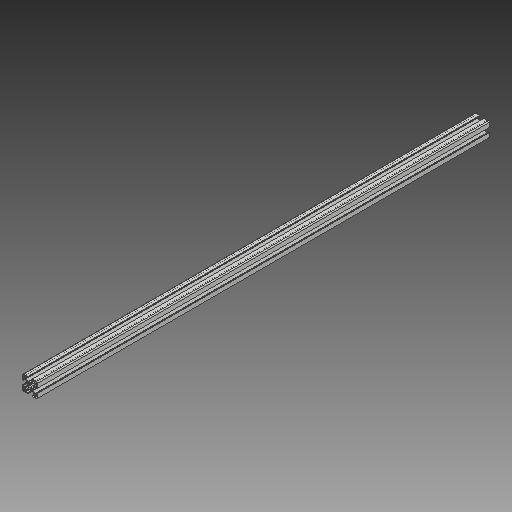
# Autodesk Inventor part: 3030 900mm_CPY
Saved by Autodesk Inventor 2018 (Build 220112000, 112)
## iProperties
Created: 2016-07-11
Part Number: 3030 900mm_CPY
Material: Generic
Document SubType Name: Modeling
Designer: joshmamo
Density: 1 g/cm^3
Appearance: Default
Author: joshm
Autodesk Inventor part; units mm, degrees
ref_plane "YZ Plane" through (0, 0, 0) normal (1, 0, 0) x (0, 1, 0)
ref_plane "XZ Plane" through (0, 0, 0) normal (0, 1, 0) x (-1, 0, 0)
ref_plane "XY Plane" through (0, 0, 0) normal (0, 0, 1) x (1, 0, 0)
sketch "Sketch1" plane through (0, 0, 0) normal (0, 0, 1) x (1, 0, 0)
  line L0 (-2.4733, -3.9798) -> (-1.4942, -3.198) projected
  arc A0 (-1.4942, -3.198) -> (1.4942, -3.198) centre (0, 0.0001) ccw projected
  line L1 (1.4942, -3.198) -> (2.4733, -3.9798) projected
  arc A1 (2.4733, -3.9798) -> (3.9799, -2.4732) centre (3.1422, -3.1421) ccw projected
  line L2 (3.9799, -2.4732) -> (3.1981, -1.4941) projected
  arc A2 (3.1981, -1.4941) -> (3.1981, 1.4944) centre (0, 0.0001) ccw projected
  line L3 (3.1981, 1.4944) -> (3.9799, 2.4735) projected
  arc A3 (3.9799, 2.4735) -> (2.4733, 3.9801) centre (3.1422, 3.1424) ccw projected
  line L4 (2.4733, 3.9801) -> (1.4942, 3.1983) projected
  arc A4 (1.4942, 3.1983) -> (-1.4942, 3.1983) centre (0, 0.0001) ccw projected
  line L5 (-1.4942, 3.1983) -> (-2.4733, 3.9801) projected
  arc A5 (-2.4733, 3.9801) -> (-3.9799, 2.4735) centre (-3.1422, 3.1424) ccw projected
  line L6 (-3.9799, 2.4735) -> (-3.1981, 1.4944) projected
  arc A6 (-3.1981, 1.4944) -> (-3.1981, -1.4941) centre (0, 0.0001) ccw projected
  line L7 (-3.1981, -1.4941) -> (-3.9799, -2.4732) projected
  arc A7 (-3.9799, -2.4732) -> (-2.4733, -3.9798) centre (-3.1422, -3.1421) ccw projected
  line L8 (13.3189, -9.4998) -> (9.88, -9.4998) projected
  arc A8 (9.88, -9.4998) -> (9.5, -9.8798) centre (9.88, -9.8798) ccw projected
  line L9 (9.5, -9.8798) -> (9.5, -13.3188) projected
  arc A9 (9.5, -13.3188) -> (9.881, -13.6998) centre (9.881, -13.3188) ccw projected
  line L10 (9.881, -13.6998) -> (12.6999, -13.6998) projected
  arc A10 (12.6999, -13.6998) -> (13.6999, -12.6998) centre (12.6999, -12.6998) ccw projected
  line L11 (13.6999, -12.6998) -> (13.6999, -9.8808) projected
  arc A11 (13.6999, -9.8808) -> (13.3189, -9.4998) centre (13.3189, -9.8808) ccw projected
  line L12 (-9.5, -13.3188) -> (-9.5, -9.8798) projected
  arc A12 (-9.5, -9.8798) -> (-9.88, -9.4998) centre (-9.88, -9.8798) ccw projected
  line L13 (-9.88, -9.4998) -> (-13.3189, -9.4998) projected
  arc A13 (-13.3189, -9.4998) -> (-13.6999, -9.8808) centre (-13.3189, -9.8808) ccw projected
  line L14 (-13.6999, -9.8808) -> (-13.6999, -12.6998) projected
  arc A14 (-13.6999, -12.6998) -> (-12.6999, -13.6998) centre (-12.6999, -12.6998) ccw projected
  line L15 (-12.6999, -13.6998) -> (-9.881, -13.6998) projected
  arc A15 (-9.881, -13.6998) -> (-9.5, -13.3188) centre (-9.881, -13.3188) ccw projected
  line L16 (-13.3189, 9.5001) -> (-9.88, 9.5001) projected
  arc A16 (-9.88, 9.5001) -> (-9.5, 9.8801) centre (-9.88, 9.8801) ccw projected
  line L17 (-9.5, 9.8801) -> (-9.5, 13.3191) projected
  arc A17 (-9.5, 13.3191) -> (-9.881, 13.7001) centre (-9.881, 13.3191) ccw projected
  line L18 (-9.881, 13.7001) -> (-12.6999, 13.7001) projected
  arc A18 (-12.6999, 13.7001) -> (-13.6999, 12.7001) centre (-12.6999, 12.7001) ccw projected
  line L19 (-13.6999, 12.7001) -> (-13.6999, 9.8811) projected
  arc A19 (-13.6999, 9.8811) -> (-13.3189, 9.5001) centre (-13.3189, 9.8811) ccw projected
  line L20 (9.5, 13.3191) -> (9.5, 9.8801) projected
  arc A20 (9.5, 9.8801) -> (9.88, 9.5001) centre (9.88, 9.8801) ccw projected
  line L21 (9.88, 9.5001) -> (13.3189, 9.5001) projected
  arc A21 (13.3189, 9.5001) -> (13.6999, 9.8811) centre (13.3189, 9.8811) ccw projected
  line L22 (13.6999, 9.8811) -> (13.6999, 12.7001) projected
  arc A22 (13.6999, 12.7001) -> (12.6999, 13.7001) centre (12.6999, 12.7001) ccw projected
  line L23 (12.6999, 13.7001) -> (9.881, 13.7001) projected
  arc A23 (9.881, 13.7001) -> (9.5, 13.3191) centre (9.881, 13.3191) ccw projected
  arc A24 (4, 13.2426) -> (4.5, 12.7426) centre (4.5, 13.2426) ccw projected
  line L24 (4, 13.2426) -> (4, 14.5001) projected
  arc A25 (4.5, 15.0001) -> (4, 14.5001) centre (4.5, 14.5001) ccw projected
  line L25 (4.5, 15.0001) -> (12.9999, 15.0001) projected
  arc A26 (14.9999, 13.0001) -> (12.9999, 15.0001) centre (12.9999, 13.0001) ccw projected
  line L26 (14.9999, 13.0001) -> (14.9999, 4.5001) projected
  arc A27 (14.4999, 4.0001) -> (14.9999, 4.5001) centre (14.4999, 4.5001) ccw projected
  line L27 (14.4999, 4.0001) -> (13.2425, 4.0001) projected
  arc A28 (12.7425, 4.5001) -> (13.2425, 4.0001) centre (13.2425, 4.5001) ccw projected
  line L28 (12.7425, 4.5001) -> (12.7425, 7.7327) projected
  arc A29 (12.7425, 7.7327) -> (12.2428, 8.2501) centre (12.2428, 7.7501) ccw projected
  line L29 (12.2428, 8.2501) -> (10.2602, 8.2501) projected
  arc A30 (10.2602, 8.2501) -> (9.9066, 8.1037) centre (10.2602, 7.7501) ccw projected
  line L30 (9.9066, 8.1037) -> (5.9811, 4.1781) projected
  arc A31 (5.9811, 4.1781) -> (5.8347, 3.8246) centre (6.3347, 3.8246) ccw projected
  line L31 (5.8347, 3.8246) -> (5.8347, 0.8876) projected
  line L32 (5.8347, 0.8876) -> (5.3247, -0.0624) projected
  line L33 (5.3247, -0.0624) -> (5.8347, -1.0124) projected
  line L34 (5.8347, -1.0124) -> (5.8347, -3.8243) projected
  arc A32 (5.8347, -3.8243) -> (5.9811, -4.1779) centre (6.3347, -3.8243) ccw projected
  line L35 (5.9811, -4.1779) -> (9.9066, -8.1034) projected
  arc A33 (9.9066, -8.1034) -> (10.2602, -8.2498) centre (10.2602, -7.7498) ccw projected
  line L36 (10.2602, -8.2498) -> (12.2428, -8.2498) projected
  arc A34 (12.2428, -8.2498) -> (12.7425, -7.7324) centre (12.2428, -7.7498) ccw projected
  line L37 (12.7425, -7.7324) -> (12.7425, -4.4999) projected
  arc A35 (13.2425, -3.9999) -> (12.7425, -4.4999) centre (13.2425, -4.4999) ccw projected
  line L38 (13.2425, -3.9999) -> (14.4999, -3.9999) projected
  arc A36 (14.9999, -4.4999) -> (14.4999, -3.9999) centre (14.4999, -4.4999) ccw projected
  line L39 (14.9999, -4.4999) -> (14.9999, -12.9998) projected
  arc A37 (12.9999, -14.9998) -> (14.9999, -12.9998) centre (12.9999, -12.9998) ccw projected
  line L40 (12.9999, -14.9998) -> (4.5, -14.9998) projected
  arc A38 (4, -14.4998) -> (4.5, -14.9998) centre (4.5, -14.4998) ccw projected
  line L41 (4, -14.4998) -> (4, -13.2423) projected
  arc A39 (4.5, -12.7423) -> (4, -13.2423) centre (4.5, -13.2423) ccw projected
  line L42 (4.5, -12.7423) -> (7.7325, -12.7423) projected
  arc A40 (7.7325, -12.7423) -> (8.25, -12.2426) centre (7.75, -12.2426) ccw projected
  line L43 (8.25, -12.2426) -> (8.25, -10.26) projected
  arc A41 (8.25, -10.26) -> (8.1035, -9.9065) centre (7.75, -10.26) ccw projected
  line L44 (8.1035, -9.9065) -> (4.178, -5.981) projected
  arc A42 (4.178, -5.981) -> (3.8245, -5.8345) centre (3.8245, -6.3345) ccw projected
  line L45 (3.8245, -5.8345) -> (0.95, -5.8345) projected
  line L46 (0.95, -5.8345) -> (0, -5.3245) projected
  line L47 (0, -5.3245) -> (-0.95, -5.8345) projected
  line L48 (-0.95, -5.8345) -> (-3.8245, -5.8345) projected
  arc A43 (-3.8245, -5.8345) -> (-4.178, -5.981) centre (-3.8245, -6.3345) ccw projected
  line L49 (-4.178, -5.981) -> (-8.1035, -9.9065) projected
  arc A44 (-8.1035, -9.9065) -> (-8.25, -10.26) centre (-7.75, -10.26) ccw projected
  line L50 (-8.25, -10.26) -> (-8.25, -12.2426) projected
  arc A45 (-8.25, -12.2426) -> (-7.7325, -12.7423) centre (-7.75, -12.2426) ccw projected
  line L51 (-7.7325, -12.7423) -> (-4.5, -12.7423) projected
  arc A46 (-4, -13.2423) -> (-4.5, -12.7423) centre (-4.5, -13.2423) ccw projected
  line L52 (-4, -13.2423) -> (-4, -14.4998) projected
  arc A47 (-4.5, -14.9998) -> (-4, -14.4998) centre (-4.5, -14.4998) ccw projected
  line L53 (-4.5, -14.9998) -> (-12.9999, -14.9998) projected
  arc A48 (-14.9999, -12.9998) -> (-12.9999, -14.9998) centre (-12.9999, -12.9998) ccw projected
  line L54 (-14.9999, -12.9998) -> (-14.9999, -4.4999) projected
  arc A49 (-14.4999, -3.9999) -> (-14.9999, -4.4999) centre (-14.4999, -4.4999) ccw projected
  line L55 (-14.4999, -3.9999) -> (-13.2425, -3.9999) projected
  arc A50 (-12.7425, -4.4999) -> (-13.2425, -3.9999) centre (-13.2425, -4.4999) ccw projected
  line L56 (-12.7425, -4.4999) -> (-12.7425, -7.7324) projected
  arc A51 (-12.7425, -7.7324) -> (-12.2428, -8.2498) centre (-12.2428, -7.7498) ccw projected
  line L57 (-12.2428, -8.2498) -> (-10.2602, -8.2498) projected
  arc A52 (-10.2602, -8.2498) -> (-9.9066, -8.1034) centre (-10.2602, -7.7498) ccw projected
  line L58 (-9.9066, -8.1034) -> (-5.9811, -4.1779) projected
  arc A53 (-5.9811, -4.1779) -> (-5.8347, -3.8243) centre (-6.3347, -3.8243) ccw projected
  line L59 (-5.8347, -3.8243) -> (-5.8347, -1.0124) projected
  line L60 (-5.8347, -1.0124) -> (-5.3247, -0.0624) projected
  line L61 (-5.3247, -0.0624) -> (-5.8347, 0.8876) projected
  line L62 (-5.8347, 0.8876) -> (-5.8347, 3.8246) projected
  arc A54 (-5.8347, 3.8246) -> (-5.9811, 4.1781) centre (-6.3347, 3.8246) ccw projected
  line L63 (-5.9811, 4.1781) -> (-9.9066, 8.1037) projected
  arc A55 (-9.9066, 8.1037) -> (-10.2602, 8.2501) centre (-10.2602, 7.7501) ccw projected
  line L64 (-10.2602, 8.2501) -> (-12.2428, 8.2501) projected
  arc A56 (-12.2428, 8.2501) -> (-12.7425, 7.7327) centre (-12.2428, 7.7501) ccw projected
  line L65 (-12.7425, 7.7327) -> (-12.7425, 4.5001) projected
  arc A57 (-13.2425, 4.0001) -> (-12.7425, 4.5001) centre (-13.2425, 4.5001) ccw projected
  line L66 (-13.2425, 4.0001) -> (-14.4999, 4.0001) projected
  arc A58 (-14.9999, 4.5001) -> (-14.4999, 4.0001) centre (-14.4999, 4.5001) ccw projected
  line L67 (-14.9999, 4.5001) -> (-14.9999, 13.0001) projected
  arc A59 (-12.9999, 15.0001) -> (-14.9999, 13.0001) centre (-12.9999, 13.0001) ccw projected
  line L68 (-12.9999, 15.0001) -> (-4.5, 15.0001) projected
  arc A60 (-4, 14.5001) -> (-4.5, 15.0001) centre (-4.5, 14.5001) ccw projected
  line L69 (-4, 14.5001) -> (-4, 13.2426) projected
  arc A61 (-4.5, 12.7426) -> (-4, 13.2426) centre (-4.5, 13.2426) ccw projected
  line L70 (-4.5, 12.7426) -> (-7.7325, 12.7426) projected
  arc A62 (-7.7325, 12.7426) -> (-8.25, 12.2429) centre (-7.75, 12.2429) ccw projected
  line L71 (-8.25, 12.2429) -> (-8.25, 10.2603) projected
  arc A63 (-8.25, 10.2603) -> (-8.1035, 9.9068) centre (-7.75, 10.2603) ccw projected
  line L72 (-8.1035, 9.9068) -> (-4.178, 5.9813) projected
  arc A64 (-4.178, 5.9813) -> (-3.8245, 5.8348) centre (-3.8245, 6.3348) ccw projected
  line L73 (-3.8245, 5.8348) -> (-0.95, 5.8348) projected
  line L74 (-0.95, 5.8348) -> (0, 5.3248) projected
  line L75 (0, 5.3248) -> (0.95, 5.8348) projected
  line L76 (0.95, 5.8348) -> (3.8245, 5.8348) projected
  arc A65 (3.8245, 5.8348) -> (4.178, 5.9813) centre (3.8245, 6.3348) ccw projected
  line L77 (4.178, 5.9813) -> (8.1035, 9.9068) projected
  arc A66 (8.1035, 9.9068) -> (8.25, 10.2603) centre (7.75, 10.2603) ccw projected
  line L78 (8.25, 10.2603) -> (8.25, 12.2429) projected
  arc A67 (8.25, 12.2429) -> (7.7325, 12.7426) centre (7.75, 12.2429) ccw projected
  line L79 (7.7325, 12.7426) -> (4.5, 12.7426) projected
  point P0 (0, 0)
extrude "Extrusion1" add sketch "Sketch1" along normal blind 900
body "Solid1"
